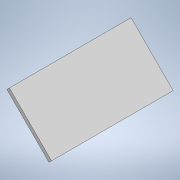
# Autodesk Inventor part: lustro
Saved by Autodesk Inventor 2022 (Build 260153000, 153)
## iProperties
Created: 2022-12-26
Part Number: lustro
Material: Generic
Document SubType Name: Modeling
Designer: Kamil
Density: 1 g/cm^3
Appearance: Default
Author: Kamil
Autodesk Inventor part; units mm, degrees
ref_plane "YZ Plane" through (0, 0, 0) normal (1, 0, 0) x (0, 1, 0)
ref_plane "XZ Plane" through (0, 0, 0) normal (0, 1, 0) x (-1, 0, 0)
sketch "Sketch1" plane through (0, 0, 0) normal (0, 0, 1) x (1, 0, 0)
  line L0 (-46.3287, 13.05) -> (-28.2287, 13.05) projected
  arc A0 (-10.1287, -5.05) -> (-28.2287, 13.05) centre (-28.2287, -5.05) ccw projected
  line L1 (-10.1287, -5.05) -> (-10.1287, -16.05) projected
  line L2 (-10.1287, -16.05) -> (46.3287, -16.05) projected
  line L3 (46.3287, -16.05) -> (14.2287, 16.05) projected
  line L4 (14.2287, 16.05) -> (-46.3287, 16.05) projected
  line L5 (-46.3287, 16.05) -> (-46.3287, 13.05) projected
  line L6 (40.8221, -6.3008) -> (55.6713, -21.15) projected
  line L7 (38.7008, -8.4221) -> (40.8221, -6.3008) projected
  line L8 (51.4287, -21.15) -> (38.7008, -8.4221) projected
  line L9 (55.6713, -21.15) -> (51.4287, -21.15) projected
  line L10 (40.8221, -6.3008) -> (12.5545, 21.9669)
  line L11 (12.5545, 21.9669) -> (6.2038, 28.3175)
  line L12 (6.2038, 28.3175) -> (4.0825, 26.1962)
  line L13 (4.0825, 26.1962) -> (38.7008, -8.4221)
  point P0 (0, 0)
  point P1 (14.2287, 16.05)
  constraints: 8 end point, 1 collinear, 1 perpendicular, 1 point on line
ref_plane "Work Plane1" through (-10.1287, -19.05, -100) normal (0, 0, -1) x (0, 1, 0)
extrude "Extrusion1" add sketch "Sketch1" against normal up to surface (100 mm away) contours L13 L12 L11 L10 L7 L3
body "Solid1"
